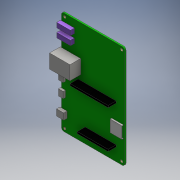
# Autodesk Inventor part: STM32F746G-Disco
Saved by Autodesk Inventor 2016 SP1 (Build 200210100, 210)
## iProperties
Created: 2018-06-05
Part Number: STM32F746G-Disco
Material: Générique
Document SubType Name: Modeling
Designer: dimercur
Density: 1 g/cm^3
Appearance: Par défaut
Author: dimercur
Autodesk Inventor part; units mm, degrees
ref_plane "YZ Plane" through (0, 0, 0) normal (1, 0, 0) x (0, 1, 0)
ref_plane "XZ Plane" through (0, 0, 0) normal (0, 1, 0) x (-1, 0, 0)
ref_plane "XY Plane" through (0, 0, 0) normal (0, 0, 1) x (1, 0, 0)
sketch "Esquisse1" plane through (0, 0, 0) normal (0, 1, 0) x (-1, 0, 0)
  line L0 (40, 65) -> (-40, 65)
  line L1 (-40, 65) -> (-40, -65)
  line L2 (-40, -65) -> (40, -65)
  line L3 (40, -65) -> (40, 65)
  point P0 (0, 0)
  dimension "d0" = 130
  dimension "d1" = 80
  dimension "d2" = 40
  dimension "d3" = 65
  constraints: 8 end point, 2 parallel, 1 horizontal, 1 perpendicular
  measures "d0" distance of L2.end L0.start
  measures "d1" distance of L0.start L0.end
  measures "d2" horizontal distance of point (0, 0) L0.start
  measures "d3" vertical distance of point (0, 0) L0.start
extrude "Extrusion1" add sketch "Esquisse1" along normal blind 1.6
sketch "Esquisse2" plane through (0, 1.6, 0) normal (0, 1, 0) x (1, 0, 0)
  circle A0 centre (-36, -61) radius 1.6
  circle A1 centre (-36, 61) radius 1.6
  circle A2 centre (36, 61) radius 1.6
  circle A3 centre (36, -61) radius 1.6
  point P0 (0, 0)
  dimension "d6" = 3.2
  dimension "d7" = 3.2
  dimension "d8" = 3.2
  dimension "d9" = 3.2
  dimension "d10" = 122
  dimension "d11" = 122
  dimension "d12" = 72
  dimension "d13" = 72
  dimension "d14" = 61
  dimension "d15" = 36
  dimension "d16" = 36
  dimension "d17" = 61
  constraints: 4 centre point
  measures "d6" diameter of A0
  measures "d7" diameter of A1
  measures "d8" diameter of A2
  measures "d9" diameter of A3
  measures "d10" distance of A1.centre A0.centre
  measures "d11" distance of A2.centre A3.centre
  measures "d12" distance of A0.centre A3.centre
  measures "d13" distance of A2.centre A1.centre
  measures "d14" vertical distance of point (0, 0) A0.centre
  measures "d15" horizontal distance of point (0, 0) A1.centre
  measures "d16" horizontal distance of point (0, 0) A0.centre
  measures "d17" vertical distance of A3.centre point (0, 0)
extrude "Extrusion2" cut sketch "Esquisse2" against normal blind 1.6
fillet "Congé1" radius 3.2 4 edges at (-40, 0.8, 65) (40, 0.8, 65) (40, 0.8, -65) (-40, 0.8, -65)
sketch "Esquisse3" plane through (0, 1.6, 0) normal (0, 1, 0) x (1, 0, 0)
  line L0 (-35, -53) -> (33, -53)
  line L1 (33, -53) -> (33, 53)
  line L2 (33, 53) -> (-35, 53)
  line L3 (-35, 53) -> (-35, -53)
  line L4 (40, -61.8) -> (40, 61.8) projected
  line L5 (36.8, 65) -> (-36.8, 65) projected
  point P0 (0, 0)
  dimension "d21" = 106
  dimension "d22" = 68
  dimension "d23" = 7
  dimension "d24" = 12
  constraints: 8 end point, 2 parallel, 1 horizontal, 1 perpendicular
  measures "d21" distance of L2.end L0.start
  measures "d22" distance of L1.end L2.end
  measures "d23" distance between parallel lines of L4 L1
  measures "d24" distance between parallel lines of L5 L2
extrude "Extrusion3" add sketch "Esquisse3" along normal blind 6
sketch "Esquisse4" plane through (0, 1.6, 0) normal (0, 1, 0) x (1, 0, 0)
  line L0 (-12.5, -59) -> (-8.5, -59)
  line L1 (-8.5, -59) -> (-8.5, -62)
  line L2 (-8.5, -62) -> (-12.5, -62)
  line L3 (-12.5, -62) -> (-12.5, -59)
  line L4 (8.5, -59) -> (12.5, -59)
  line L5 (12.5, -59) -> (12.5, -62)
  line L6 (12.5, -62) -> (8.5, -62)
  line L7 (8.5, -62) -> (8.5, -59)
  line L8 (-36.8, -65) -> (36.8, -65) projected
  line L9 (40, -61.8) -> (40, 61.8) projected
  point P0 (0, 0)
  dimension "d27" = 4
  dimension "d28" = 3
  dimension "d29" = 6
  dimension "d30" = 6
  dimension "d31" = 4
  dimension "d32" = 17
  dimension "d33" = 27.5
  constraints: 16 end point, 4 parallel, 2 horizontal, 2 perpendicular, 1 point on line
  measures "d27" distance of L0.start L0.end
  measures "d28" distance between parallel lines of L8 L2
  measures "d29" distance between parallel lines of L8 L0
  measures "d30" distance between parallel lines of L8 L4
  measures "d31" distance between parallel lines of L5 L7
  measures "d32" distance between parallel lines of L7 L1
  measures "d33" distance between parallel lines of L9 L5
extrude "Extrusion4" add sketch "Esquisse4" along normal blind 1
sketch "Esquisse5" plane through (0, 0, 0) normal (0, -1, 0) x (1, 0, 0)
  line L0 (-41.9, -48.5) -> (-32.9, -48.5)
  line L1 (-32.9, -48.5) -> (-32.9, -40.5)
  line L2 (-32.9, -40.5) -> (-41.9, -40.5)
  line L3 (-41.9, -40.5) -> (-41.9, -48.5)
  line L4 (36.8, -65) -> (-36.8, -65) projected
  line L5 (-40, -61.8) -> (-40, 61.8) projected
  point P0 (0, 0)
  dimension "d36" = 8
  dimension "d37" = 9
  dimension "d38" = 16.5
  dimension "d39" = 1.9
  constraints: 8 end point, 2 parallel, 1 horizontal, 1 perpendicular
  measures "d36" distance between parallel lines of L2 L0
  measures "d37" distance between parallel lines of L1 L3
  measures "d38" distance between parallel lines of L4 L0
  measures "d39" distance between parallel lines of L5 L3
extrude "Extrusion5" add sketch "Esquisse5" along normal blind 4.2
sketch "Esquisse6" plane through (0, 0, 0) normal (0, -1, 0) x (1, 0, 0)
  line L0 (-35, 53) -> (-35, -53) projected
  line L1 (-41, -26.7) -> (-35, -26.7)
  line L2 (-35, -26.7) -> (-35, -18.7)
  line L3 (-35, -18.7) -> (-41, -18.7)
  line L4 (-41, -18.7) -> (-41, -26.7)
  line L5 (-41, -9.1) -> (-35, -9.1)
  line L6 (-35, -9.1) -> (-35, -1.1)
  line L7 (-35, -1.1) -> (-41, -1.1)
  line L8 (-41, -1.1) -> (-41, -9.1)
  line L9 (-32.9, -40.5) -> (-41.9, -40.5) projected
  line L10 (-40, -61.8) -> (-40, 61.8) projected
  point P0 (0, 0)
  dimension "d42" = 8
  dimension "d43" = 8
  dimension "d44" = 6
  dimension "d45" = 13.8
  dimension "d46" = 9.6
  dimension "d47" = 1
  constraints: 16 end point, 4 parallel, 3 point on line, 2 horizontal, 2 perpendicular
  measures "d42" distance between parallel lines of L3 L1
  measures "d43" distance between parallel lines of L7 L5
  measures "d44" distance between parallel lines of L0 L4
  measures "d45" distance between parallel lines of L9 L1
  measures "d46" distance between parallel lines of L5 L3
  measures "d47" distance between parallel lines of L10 L4
extrude "Extrusion6" add sketch "Esquisse6" along normal blind 2.8 contours L0 L5 L10 L7 | L10 L5 L8 L7 | L0 L1 L10 L3 | L10 L1 L4 L3
sketch "Esquisse7" plane through (0, 0, 0) normal (0, -1, 0) x (1, 0, 0)
  line L0 (-41.4, 7.9) -> (-15.7, 7.9)
  line L1 (-15.7, 7.9) -> (-15.7, 25.6)
  line L2 (-15.7, 25.6) -> (-41.4, 25.6)
  line L3 (-41.4, 25.6) -> (-41.4, 7.9)
  line L4 (-35, -1.1) -> (-41, -1.1) projected
  line L5 (-40, -1.1) -> (-40, 61.8) projected
  point P0 (0, 0)
  dimension "d50" = 25.7
  dimension "d51" = 17.7
  dimension "d52" = 9
  dimension "d53" = 1.4
  constraints: 8 end point, 2 parallel, 1 horizontal, 1 perpendicular
  measures "d50" distance between parallel lines of L1 L3
  measures "d51" distance between parallel lines of L2 L0
  measures "d52" distance between parallel lines of L0 L4
  measures "d53" distance between parallel lines of L5 L3
extrude "Extrusion7" add sketch "Esquisse7" along normal blind 13.6
sketch "Esquisse8" plane through (0, 0, 0) normal (0, -1, 0) x (1, 0, 0)
  line L0 (-41, 38) -> (-23.6, 38)
  line L1 (-23.6, 38) -> (-23.6, 44)
  line L2 (-23.6, 44) -> (-41, 44)
  line L3 (-41, 44) -> (-41, 38)
  line L4 (-41, 49) -> (-23.6, 49)
  line L5 (-23.6, 49) -> (-23.6, 55)
  line L6 (-23.6, 55) -> (-41, 55)
  line L7 (-41, 55) -> (-41, 49)
  line L8 (-15.7, 25.6) -> (-41.4, 25.6) projected
  line L9 (-40, 25.6) -> (-40, 61.8) projected
  point P0 (0, 0)
  dimension "d56" = 6
  dimension "d57" = 6
  dimension "d58" = 17.4
  dimension "d59" = 5
  dimension "d60" = 12.4
  dimension "d61" = 1
  constraints: 16 end point, 4 parallel, 2 horizontal, 2 perpendicular, 2 point on line
  measures "d56" distance between parallel lines of L2 L0
  measures "d57" distance between parallel lines of L6 L4
  measures "d58" distance between parallel lines of L1 L3
  measures "d59" distance between parallel lines of L4 L2
  measures "d60" distance between parallel lines of L0 L8
  measures "d61" distance between parallel lines of L9 L3
extrude "Extrusion8" add sketch "Esquisse8" along normal blind 5
sketch "Esquisse9" plane through (-41.4, 0, 7.9) normal (-1, 0, 0) x (0, 0, 1)
  line L0 (2.85, -2.2) -> (14.85, -2.2)
  line L1 (14.85, -2.2) -> (14.85, -9.2)
  line L2 (14.85, -9.2) -> (2.85, -9.2)
  line L3 (2.85, -9.2) -> (2.85, -2.2)
  line L4 (17.7, 0) -> (0, 0) projected
  line L5 (17.7, 0) -> (17.7, -13.6) projected
  line L6 (0, 0) -> (0, -13.6) projected
  point P0 (-7.9, 0)
  dimension "d64" = 12
  dimension "d65" = 7
  dimension "d66" = 2.2
  dimension "d67" = 17.7
  dimension "d68" = 2.85
  constraints: 8 end point, 2 parallel, 1 horizontal, 1 perpendicular
  measures "d64" distance between parallel lines of L1 L3
  measures "d65" distance between parallel lines of L2 L0
  measures "d66" distance between parallel lines of L0 L4
  measures "d67" distance between parallel lines of L5 L6
  measures "d68" distance between parallel lines of L3 L6
extrude "Extrusion9" cut sketch "Esquisse9" against normal blind 11
sketch "Esquisse10" plane through (-41.9, 0, -48.5) normal (-1, 0, 0) x (0, 0, 1)
  line L0 (1, -0.6) -> (7, -0.6)
  line L1 (7, -0.6) -> (7, -3.6)
  line L2 (7, -3.6) -> (1, -3.6)
  line L3 (1, -3.6) -> (1, -0.6)
  line L4 (22.55, -0.4) -> (29.05, -0.4)
  line L5 (29.05, -0.4) -> (29.05, -2.4)
  line L6 (29.05, -2.4) -> (22.55, -2.4)
  line L7 (22.55, -2.4) -> (22.55, -0.4)
  line L8 (40.15, -0.4) -> (46.65, -0.4)
  line L9 (46.65, -0.4) -> (46.65, -2.4)
  line L10 (46.65, -2.4) -> (40.15, -2.4)
  line L11 (40.15, -2.4) -> (40.15, -0.4)
  circle A0 centre (89.5, -2.5) radius 1.8
  circle A1 centre (100.5, -2.5) radius 1.8
  line L12 (8, 0) -> (0, 0) projected
  line L13 (8, -4.2) -> (0, -4.2) projected
  line L14 (8, 0) -> (8, -4.2) projected
  line L15 (0, 0) -> (0, -4.2) projected
  line L16 (29.8, 0) -> (21.8, 0) projected
  line L17 (29.8, -2.8) -> (21.8, -2.8) projected
  line L18 (29.8, 0) -> (29.8, -2.8) projected
  line L19 (21.8, 0) -> (21.8, -2.8) projected
  line L20 (47.4, 0) -> (47.4, -2.8) projected
  line L21 (39.4, 0) -> (39.4, -2.8) projected
  line L22 (92.5, 0) -> (92.5, -5) projected
  line L23 (86.5, 0) -> (86.5, -5) projected
  line L24 (92.5, 0) -> (86.5, 0) projected
  line L25 (92.5, -5) -> (86.5, -5) projected
  line L26 (97.5, 0) -> (97.5, -5) projected
  point P0 (48.5, 0)
  dimension "d71" = 3
  dimension "d72" = 2
  dimension "d73" = 2
  dimension "d74" = 6
  dimension "d75" = 6.5
  dimension "d76" = 6.5
  dimension "d77" = 4.2
  dimension "d78" = 8
  dimension "d79" = 2.8
  dimension "d80" = 8
  dimension "d81" = 8
  dimension "d82" = 1
  dimension "d83" = 0.6
  dimension "d84" = 0.75
  dimension "d86" = 0.4
  dimension "d87" = 0.75
  dimension "d88" = 6
  dimension "d89" = 5
  dimension "d90" = 3
  dimension "d91" = 2.5
  dimension "d92" = 3
  dimension "d93" = 2.5
  dimension "d94" = 3.6
  dimension "d95" = 3.6
  constraints: 24 end point, 6 parallel, 3 horizontal, 3 perpendicular, 2 centre point, 2 point on line
  measures "d71" distance between parallel lines of L2 L0
  measures "d72" distance between parallel lines of L6 L4
  measures "d73" distance between parallel lines of L10 L8
  measures "d74" distance between parallel lines of L1 L3
  measures "d75" distance between parallel lines of L5 L7
  measures "d76" distance between parallel lines of L9 L11
  measures "d77" distance between parallel lines of L12 L13
  measures "d78" distance between parallel lines of L14 L15
  measures "d79" distance between parallel lines of L16 L17
  measures "d80" distance between parallel lines of L18 L19
  measures "d81" distance between parallel lines of L20 L21
  measures "d82" distance between parallel lines of L15 L3
  measures "d83" distance between parallel lines of L12 L0
  measures "d84" distance between parallel lines of L19 L7
  measures "d86" distance between parallel lines of L17 L6
  measures "d87" distance between parallel lines of L21 L11
  measures "d88" distance between parallel lines of L22 L23
  measures "d89" distance between parallel lines of L24 L25
  measures "d90" distance from line of L23 A0.centre
  measures "d91" distance from line of L24 A0.centre
  measures "d92" distance from line of L26 A1.centre
  measures "d93" vertical distance of L26.start A1.centre
  measures "d94" diameter of A0
  measures "d95" diameter of A1
extrude "Extrusion10" cut sketch "Esquisse10" against normal blind 4 contours L0 L1 L2 L3 | L4 L5 L6 L7 | L8 L9 L10 L11 | A0 | A1
sketch "Esquisse11" plane through (0, 0, 0) normal (0, -1, 0) x (1, 0, 0)
  line L0 (38.5, -35) -> (23.5, -35)
  line L1 (23.5, -35) -> (23.5, -20)
  line L2 (23.5, -20) -> (38.5, -20)
  line L3 (38.5, -20) -> (38.5, -35)
  line L4 (40, 61.8) -> (40, -61.8) projected
  line L5 (36.8, -65) -> (-36.8, -65) projected
  point P0 (0, 0)
  dimension "d98" = 15
  dimension "d99" = 15
  dimension "d100" = 1.5
  dimension "d101" = 30
  constraints: 8 end point, 2 parallel, 1 horizontal, 1 perpendicular
  measures "d98" distance of L0.start L0.end
  measures "d99" distance of L0.end L1.end
  measures "d100" distance between parallel lines of L4 L3
  measures "d101" distance between parallel lines of L5 L0
extrude "Extrusion11" add sketch "Esquisse11" along normal blind 2
sketch "Esquisse13" plane through (38.5, 0, -20) normal (1, 0, 0) x (0, 0, -1)
  line L0 (-1.3, 0) -> (6.7, 0) projected
  line L1 (14.7, -1.7) -> (0.3, -1.7)
  line L2 (0.3, -1.7) -> (0.3, 0)
  line L3 (0.3, 0) -> (14.7, 0)
  line L4 (14.7, 0) -> (14.7, -1.7)
  line L5 (0, 0) -> (0, -2) projected
  line L6 (15, 0) -> (15, -2) projected
  point P0 (-20, 0)
  dimension "d104" = 0.3
  dimension "d106" = 0.3
  dimension "d107" = 0.3
  constraints: 8 end point, 2 parallel, 1 horizontal, 1 perpendicular, 1 point on line
  measures "d104" distance between parallel lines of L2 L5
  measures "d106" distance between parallel lines of L6 L4
  measures "d107" distance from line of L5.end L1
extrude "Extrusion12" cut sketch "Esquisse13" against normal blind 12
sketch "Esquisse14" plane through (0, 0, 0) normal (0, -1, 0) x (1, 0, 0)
  line L0 (-10, -49) -> (29, -49)
  line L1 (29, -49) -> (29, -46.5)
  line L2 (29, -46.5) -> (-10, -46.5)
  line L3 (-10, -46.5) -> (-10, -49)
  line L4 (-19, -1) -> (29, -1)
  line L5 (29, -1) -> (29, 1.5)
  line L6 (29, 1.5) -> (-19, 1.5)
  line L7 (-19, 1.5) -> (-19, -1)
  line L8 (40, 61.8) -> (40, -61.8) projected
  line L9 (36.8, -65) -> (-36.8, -65) projected
  point P0 (0, 0)
  dimension "d110" = 2.5
  dimension "d111" = 2.5
  dimension "d112" = 39
  dimension "d113" = 48
  dimension "d114" = 11
  dimension "d115" = 16
  dimension "d116" = 64
  constraints: 16 end point, 4 parallel, 2 horizontal, 2 perpendicular, 1 point on line
  measures "d110" distance of L2.end L0.start
  measures "d111" distance of L6.end L4.start
  measures "d112" distance of L0.start L0.end
  measures "d113" distance from line of L5.end L7
  measures "d114" distance between parallel lines of L8 L1
  measures "d115" distance between parallel lines of L9 L0
  measures "d116" distance between parallel lines of L9 L4
extrude "Extrusion13" add sketch "Esquisse14" along normal blind 10
equation "\"d2\" = 0.5 * d1"
equation "\"d3\" = 0.5 * d0"
equation "\"d14\" = 0.5 * d10"
equation "\"d15\" = 0.5 * d12"
equation "\"d16\" = 0.5 * d12"
equation "\"d17\" = 0.5 * d11"
equation "\"d31\" = d27"
equation "\"d43\" = d42"
equation "\"d57\" = d56"
equation "\"d68\" = -0.5 * d64 + 0.5 * d67"
equation "\"d82\" = -0.5 * d74 + 0.5 * d78"
equation "\"d83\" = -0.5 * d71 + 0.5 * d77"
equation "\"d84\" = -0.5 * d75 + 0.5 * d80"
equation "\"d86\" = -0.5 * d72 + 0.5 * d79"
equation "\"d87\" = -0.5 * d76 + 0.5 * d81"
equation "\"d90\" = 0.5 * d88"
equation "\"d91\" = 0.5 * d89"
equation "\"d92\" = d90"
equation "\"d93\" = d91"
equation "\"d95\" = d94"
equation "\"d106\" = d104"
equation "\"d107\" = d104"
equation "\"d111\" = d110"
